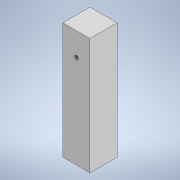
# Autodesk Inventor part: block 1
Saved by Autodesk Inventor 2021 (Build 250183000, 183)
## iProperties
Created: 2025-04-06
Part Number: block 1
Material: Generic
Document SubType Name: Modeling
Designer: Admin
Density: 1 g/cm^3
Appearance: Default
Author: Admin
Autodesk Inventor part; units mm, degrees
ref_plane "YZ Plane" through (0, 0, 0) normal (1, 0, 0) x (0, 1, 0)
ref_plane "XZ Plane" through (0, 0, 0) normal (0, 1, 0) x (-1, 0, 0)
ref_plane "XY Plane" through (0, 0, 0) normal (0, 0, 1) x (1, 0, 0)
sketch "Sketch1" plane through (0, 0, 0) normal (1, 0, 0) x (0, 1, 0)
  line L0 (12.0615, 103.4313) -> (-368.9385, 103.4313)
  line L1 (-368.9385, 103.4313) -> (-368.9385, 14.5313)
  line L2 (-368.9385, 14.5313) -> (12.0615, 14.5313)
  line L3 (12.0615, 14.5313) -> (12.0615, 103.4313)
  point P0 (0, 0)
  dimension "d0" = 381
  dimension "d1" = 88.9
  dimension "d2" = 88.9
  constraints: 8 end point, 2 parallel, 1 horizontal, 1 perpendicular
  measures "d0" distance of L2.end L1.end
  measures "d1" distance between parallel lines of L0 L2
  measures "d2" distance of L2.end L0.start
extrude "Extrusion1" add sketch "Sketch1" along normal blind 88.9
sketch "Sketch2" plane through (0, -368.9385, 14.5313) normal (0, 0, -1) x (-1, 0, 0)
  circle A0 centre (-44.45, 304.8) radius 6.35
  line L0 (0, 0) -> (0, 381) projected
  line L1 (0, 381) -> (-88.9, 381) projected
  point P0 (0, 368.9385)
  dimension "d5" = 12.7
  dimension "d6" = 44.45
  dimension "d7" = 76.2
  constraints: 1 centre point
  measures "d5" diameter of A0
  measures "d6" distance from line of L0 A0.centre
  measures "d7" distance from line of A0.centre L1
extrude "Extrusion2" cut sketch "Sketch2" against normal blind 88.9
body "Solid1"
